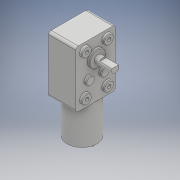
# Autodesk Inventor part: Двигатель червячный
Saved by Autodesk Inventor 2017 SP1 (Build 210196100, 196)
## iProperties
Part Number: Двигатель червячный
Material: Типовые
Document SubType Name: Modeling
Designer: sbnnl
Density: 1 g/cm^3
Appearance: По умолчанию
Author: sbnnl
Autodesk Inventor part; units mm, degrees
ref_plane "YZ Plane" through (0, 0, 0) normal (1, 0, 0) x (0, 1, 0)
ref_plane "XZ Plane" through (0, 0, 0) normal (0, 1, 0) x (-1, 0, 0)
ref_plane "XY Plane" through (0, 0, 0) normal (0, 0, 1) x (1, 0, 0)
sketch "Эскиз1" plane through (0, 0, 0) normal (1, 0, 0) x (0, 1, 0)
  line L0 (0, 0) -> (32, 0)
  line L1 (32, 0) -> (32, -46)
  line L2 (32, -46) -> (0, -46)
  line L3 (0, -46) -> (0, 0)
  dimension "d0" = 32
  dimension "d1" = 46
  constraints: 8 end point, 2 parallel, 1 horizontal, 1 perpendicular
  measures "d0" distance between parallel lines of L3 L1
  measures "d1" distance between parallel lines of L2 L0
extrude "Выдавливание1" add sketch "Эскиз1" along normal blind 22
fillet "Сопряжение1" radius 2 4 edges at (11, 32, 0) (11, 0, 0) (11, 32, -46) (11, 0, -46)
sketch "Эскиз2" plane through (0, 2, -46) normal (0, 0, -1) x (-1, 0, 0)
  circle A0 centre (-9, 16) radius 5
  line L0 (0, 30) -> (-22, 30) projected
  line L1 (-22, 0) -> (-22, 28) projected
  point P0 (0, -2)
  dimension "d5" = 10
  dimension "d6" = 14
  dimension "d7" = 13
  constraints: 1 centre point
  measures "d5" diameter of A0
  measures "d6" distance from line of A0.centre L0
  measures "d7" distance from line of L1 A0.centre
extrude "Выдавливание2" add sketch "Эскиз2" along normal blind 0.2
sketch "Эскиз3" plane through (9, 18, -46.2) normal (0, 0, -1) x (-1, 0, 0)
  circle A0 centre (0, 0) radius 5 projected
  circle A1 centre (0, 0) radius 12
  point P0 (9, -18)
  dimension "d10" = 24
  constraints: 1 centre point, 1 coincident
  measures "d10" diameter of A1
extrude "Выдавливание3" add sketch "Эскиз3" along normal blind 31 contours A0 | A1
fillet "Сопряжение2" radius 1 1 edges at (21, 18, -46.2)
sketch "Эскиз4" plane through (9, 18, -77.2) normal (0, 0, -1) x (-1, 0, 0)
  circle A0 centre (0, 0) radius 12 projected
  circle A1 centre (0, 0) radius 11.5
  circle A2 centre (0, 0) radius 3
  point P0 (9, -18)
  dimension "d14" = 0.5
  dimension "d15" = 6
  constraints: 2 centre point, 1 coincident
  measures "d14" radial gap between concentric circles of A0 A1
  measures "d15" diameter of A2
extrude "Выдавливание4" cut sketch "Эскиз4" against normal blind 1 contours A1
fillet "Сопряжение3" radius 0.3 1 edges at (12, 18, -77.2)
sketch "Эскиз5" plane through (9, 18, -76.2) normal (0, 0, -1) x (-1, 0, 0)
  circle A0 centre (0, 0) radius 2.7 projected
  circle A1 centre (0, 0) radius 2.7 projected
  circle A2 centre (0, 0) radius 3 projected
  circle A3 centre (0, 0) radius 11.5 projected
  circle A4 centre (0, 0) radius 3 projected
  line L0 (-11.4291, 0) -> (9.9709, 0) construction
  line L1 (-9.2, 1) -> (-9, 1)
  line L2 (-9, 1) -> (-9, -1)
  line L3 (-9, -1) -> (-9.2, -1)
  line L4 (-9.2, -1) -> (-9.2, 1)
  line L5 (0, 0) -> (0, 4.7597) construction
  line L6 (9.2, 1) -> (9, 1)
  line L7 (9, 1) -> (9, -1)
  line L8 (9, -1) -> (9.2, -1)
  line L9 (9.2, -1) -> (9.2, 1)
  point P0 (9, -18)
  dimension "d19" = 0.2
  dimension "d20" = 2
  dimension "d21" = 9
  constraints: 20 end point, 4 symmetric about line, 2 horizontal, 2 parallel, 1 perpendicular, 1 point on line, 1 vertical, 1 other
  measures "d19" distance between parallel lines of L2 L4
  measures "d20" distance of L1.end L2.end
  measures "d21" distance from line of A0.centre L2
extrude "Выдавливание5" add sketch "Эскиз5" along normal blind 4 contours L1 L2 L3 L4 | L9 L8 L7 L6
fillet "Сопряжение4" radius 1 4 edges at (18.1, 19, -80.2) (18.1, 17, -80.2) (-0.1, 17, -80.2) (-0.1, 19, -80.2)
sketch "Эскиз6" plane through (22, 0, 0) normal (1, 0, 0) x (0, 0, -1)
  line L0 (-9.2772, 16) -> (53.3596, 16) construction
  line L1 (44, 32) -> (2, 32) projected
  line L2 (2, 0) -> (44, 0) projected
  circle A0 centre (15, 16) radius 6.75
  line L3 (0, 30) -> (0, 2) projected
  line L4 (6, 41.4037) -> (6, -12.6668) construction
  circle A1 centre (6, 7) radius 4
  line L5 (43.6655, 7) -> (-6.8659, 7) construction
  circle A2 centre (39, 7) radius 4
  line L6 (39, 19.4288) -> (39, -2.2275) construction
  line L7 (46, 2) -> (46, 30) projected
  line L8 (28.6998, 10) -> (14.4383, 10) construction
  circle A3 centre (27.5, 10) radius 3.5
  circle A4 centre (6, 25) radius 4
  circle A5 centre (39, 25) radius 4
  line L9 (28.6998, 22) -> (14.4383, 22) construction
  circle A6 centre (27.5, 22) radius 3.5
  point P0 (0, 0)
  dimension "d25" = 32
  dimension "d26" = 16
  dimension "d27" = 13.5
  dimension "d28" = 15
  dimension "d29" = 6
  dimension "d30" = 8
  dimension "d31" = 7
  dimension "d32" = 8
  dimension "d33" = 7
  dimension "d34" = 10
  dimension "d35" = 7
  dimension "d36" = 27.5
  dimension "d60" = 9
  constraints: 12 end point, 7 centre point, 7 point on line, 5 symmetric about line, 3 horizontal, 2 vertical, 3 other
  measures "d25" distance between parallel lines of L1 L2
  measures "d26" distance between parallel lines of L0 L2
  measures "d27" diameter of A0
  measures "d28" distance from line of A0.centre L3
  measures "d29" distance between parallel lines of L4 L3
  measures "d30" diameter of A1
  measures "d31" distance between parallel lines of L5 L2
  measures "d32" diameter of A2
  measures "d33" distance between parallel lines of L6 L7
  measures "d34" distance between parallel lines of L2 L8
  measures "d35" diameter of A3
  measures "d36" distance from line of A3.centre L3
  measures "d60" distance from line of L4 A0.centre
extrude "Выдавливание6" add sketch "Эскиз6" along normal blind 2
fillet "Сопряжение5" radius 0.5 7 edges at (24, 7, -35) (24, 10, -24) (24, 16, -8.25) (24, 22, -24) (24, 25, -35) (24, 25, -2) (24, 7, -2)
sketch "Эскиз7" plane through (24, 25, -39) normal (1, 0, 0) x (0, 0, -1)
  circle A0 centre (-33, -18) radius 3.5 projected
  circle A1 centre (-33, 0) radius 3.5 projected
  circle A2 centre (-11.5, -3) radius 3 projected
  circle A3 centre (-11.5, -15) radius 3 projected
  circle A4 centre (-33, -18) radius 1.5
  circle A5 centre (-33, 0) radius 1.5
  circle A6 centre (0, -18) radius 3.5 projected
  circle A7 centre (0, 0) radius 3.5 projected
  circle A8 centre (0, -18) radius 1.5
  circle A9 centre (0, 0) radius 1.5
  circle A10 centre (-24, -9) radius 6.25 projected
  point P0 (-39, -25)
  dimension "d40" = 3
  constraints: 4 centre point, 4 coincident, 3 equal radius
  measures "d40" diameter of A4
extrude "Выдавливание7" cut sketch "Эскиз7" against normal blind 4 contours A4 | A5 | A8 | A9
sketch "Эскиз8" plane through (24, 16, -15) normal (1, 0, 0) x (0, 0, -1)
  circle A0 centre (0, 0) radius 6.25 projected
  circle A1 centre (0, 0) radius 3
  point P0 (-15, -16)
  dimension "d43" = 6
  constraints: 1 centre point, 1 coincident
  measures "d43" diameter of A1
extrude "Выдавливание8" add sketch "Эскиз8" along normal blind 14 contours A1
sketch "Эскиз9" plane through (38, 16, -15) normal (1, 0, 0) x (0, 0, -1)
  circle A0 centre (0, 0) radius 3 projected
  line L0 (-3.5, -3) -> (-1.5, -3)
  line L1 (-1.5, -3) -> (-1.5, 3)
  line L2 (-1.5, 3) -> (-3.5, 3)
  line L3 (-3.5, 3) -> (-3.5, -3)
  point P0 (-15, -16)
  dimension "d46" = 6
  dimension "d47" = 3
  dimension "d48" = 1.5
  dimension "d49" = 2
  constraints: 8 end point, 2 parallel, 1 horizontal, 1 perpendicular
  measures "d46" distance of L2.end L0.start
  measures "d47" distance from line of L0 A0.centre
  measures "d48" distance from line of L1 A0.centre
  measures "d49" distance of L1.end L2.end
extrude "Выдавливание9" cut sketch "Эскиз9" against normal blind 10 contours L1 A0 | A0 L1 L0 L3 L2 picked at (-1.9932, -0.1161)
sketch "Эскиз10" plane through (0, 0, 0) normal (-1, 0, 0) x (0, 0, 1)
  circle A0 centre (-27.5, 10) radius 3.5 projected
  circle A1 centre (-27.5, 22) radius 3.5 projected
  circle A2 centre (-15, 16) radius 3 projected
  circle A3 centre (-15, 16) radius 4
  line L0 (-33, 16) -> (-46, 16)
  line L1 (-46, 16) -> (-46, 4)
  line L2 (-46, 4) -> (-33, 4)
  line L3 (-33, 4) -> (-33, 16)
  line L4 (-46, 30) -> (-46, 2) projected
  line L5 (-2, 0) -> (-44, 0) projected
  point P0 (0, 0)
  point P1 (-46, 13.6411)
  dimension "d52" = 8
  dimension "d56" = 13
  dimension "d57" = 12
  dimension "d58" = 4
  constraints: 8 end point, 2 parallel, 1 centre point, 1 coincident, 1 collinear, 1 horizontal, 1 perpendicular
  measures "d52" diameter of A3
  measures "d56" distance of L1.end L2.end
  measures "d57" distance of L2.end L0.start
  measures "d58" distance between parallel lines of L5 L2
extrude "Выдавливание10" add sketch "Эскиз10" along normal blind 2 contours A0 | A1 | A2 | A3 | L3 L2 L1 L0
fillet "Сопряжение6" radius 0.5 7 edges at (-2, 22, -31) (-2, 10, -31) (-2, 16, -19) (-2, 4, -39.5) (-2, 10, -33) (-2, 16, -39.5) (-2, 10, -46)
fillet "Сопряжение7" radius 1 8 edges at (-1.8536, 4.1464, -33.1464) (-0.75, 4, -33) (-1.8536, 4.1464, -45.8536) (-0.75, 4, -46) (-1.8536, 15.8536, -45.8536) (-0.75, 16, -46) (-1.8536, 15.8536, -33.1464) (-0.75, 16, -33)
equation "\"d26\" = 0.5 * d25"
